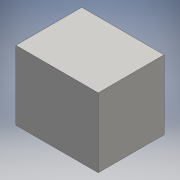
# Autodesk Inventor part: Riser
Saved by Autodesk Inventor 2016 (Build 200138000, 138)
## iProperties
Created: 2016-05-08
Part Number: Riser
Material: Generic
Document SubType Name: Modeling
Designer: Kenneth Daniel
Density: 1 g/cm^3
Appearance: Default
Author: Kenneth Daniel
Autodesk Inventor part; units mm, degrees
ref_plane "YZ Plane" through (0, 0, 0) normal (1, 0, 0) x (0, 1, 0)
ref_plane "XZ Plane" through (0, 0, 0) normal (0, 1, 0) x (-1, 0, 0)
ref_plane "XY Plane" through (0, 0, 0) normal (0, 0, 1) x (1, 0, 0)
sketch "Sketch1" plane through (0, 0, 0) normal (0, 1, 0) x (-1, 0, 0)
  line L0 (-12.5, 10.5) -> (-12.5, -10.5)
  line L1 (-12.5, -10.5) -> (12.5, -10.5)
  line L2 (12.5, -10.5) -> (12.5, 10.5)
  line L3 (12.5, 10.5) -> (-12.5, 10.5)
  line L4 (-12.5, 10.5) -> (12.5, -10.5) construction
  line L5 (-12.5, -10.5) -> (12.5, 10.5) construction
  point P0 (0, 0)
  dimension "d0" = 21
  dimension "d1" = 25
  constraints: 12 end point, 2 midpoint, 2 parallel, 1 perpendicular, 1 vertical
  measures "d0" distance of L0.start L0.end
  measures "d1" distance of L1.end L0.end
extrude "Extrusion1" add sketch "Sketch1" along normal blind 20
ref_plane "Work Plane1" through (0, 10, 0) normal (0, -1, 0) x (1, 0, 0)
ref_plane "Work Plane2" through (0, 0, -10.5) normal (-1, 0, 0) x (0, 0, 1)
ref_plane "Work Plane3" through (-12.5, 0, 0) normal (0, 0, 1) x (1, 0, 0)
body "Solid1"
